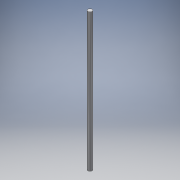
# Autodesk Inventor part: 12 mm Z rør
Saved by Autodesk Inventor 2016 (Build 200138000, 138)
## iProperties
Created: 2015-05-11
Part Number: 12 mm Z rør
Material: Aluminum 6061
Document SubType Name: Modeling
Designer: Mathias Lyngklip Kjeldgaard
Density: 2.71 g/cm^3
Appearance: Aluminum - Polished
Mass: 109.112 g
Surface Area: 136.471 cm^2
Volume: 40.2627 cm^3
Author: Mathias Lyngklip Kjeldgaard
Autodesk Inventor part; units mm, degrees
ref_plane "YZ Plane" through (0, 0, 0) normal (1, 0, 0) x (0, 1, 0)
ref_plane "XZ Plane" through (0, 0, 0) normal (0, 1, 0) x (-1, 0, 0)
ref_plane "XY Plane" through (0, 0, 0) normal (0, 0, 1) x (1, 0, 0)
sketch "Sketch1" plane through (0, 0, 0) normal (0, 0, 1) x (1, 0, 0)
  circle A0 centre (0, 0) radius 6
  dimension "d0" = 12
  constraints: 1 centre point, 1 coincident
  measures "d0" diameter of A0
extrude "Længde" add sketch "Sketch1" along normal mid plane 406
body "Solid1"
